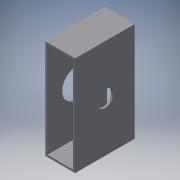
# Autodesk Inventor part: transmition Axle Support
Saved by Autodesk Inventor 2019 (Build 230136000, 136)
## iProperties
Created: 2019-10-21
Part Number: transmition Axle Support
Material: Generic
Document SubType Name: Modeling
Designer: admin
Density: 1 g/cm^3
Appearance: Default
Author: admin
Autodesk Inventor part; units mm, degrees
ref_plane "YZ Plane" through (0, 0, 0) normal (1, 0, 0) x (0, 1, 0)
ref_plane "XZ Plane" through (0, 0, 0) normal (0, 1, 0) x (-1, 0, 0)
ref_plane "XY Plane" through (0, 0, 0) normal (0, 0, 1) x (1, 0, 0)
sketch "Sketch1" plane through (0, 0, 0) normal (0, 0, 1) x (1, 0, 0)
  line L0 (-15, -50) -> (15, -50)
  line L1 (15, -50) -> (15, 50)
  line L2 (15, 50) -> (-15, 50)
  line L3 (-15, 50) -> (-15, -50)
  line L4 (-15, -50) -> (15, 50) construction
  line L5 (15, -50) -> (-15, 50) construction
  line L6 (-13, 48) -> (13, 48)
  line L7 (13, 48) -> (13, -48)
  line L8 (13, -48) -> (-13, -48)
  line L9 (-13, -48) -> (-13, 48)
  point P0 (0, 0)
  dimension "d0" = 30
  dimension "d1" = 100
  dimension "d2" = 2
  constraints: 20 end point, 4 parallel, 2 midpoint, 2 perpendicular, 1 horizontal, 3 other
  measures "d0" distance of L2.end L1.end
  measures "d1" distance of L1.end L0.end
  measures "d2" distance between parallel lines of L2 L6
extrude "Extrusion1" add sketch "Sketch1" along normal blind 60
sketch "Sketch2" plane through (15, -50, 0) normal (1, 0, 0) x (0, 0, -1)
  circle A0 centre (-30, 50) radius 8.3
  line L0 (-30, 100) -> (-30, 50) construction
  line L1 (0, 0) -> (0, 100) projected
  line L2 (0, 100) -> (-60, 100) projected
  line L3 (-30, 50) -> (0, 50) construction
  dimension "d5" = 16.6
  dimension "d11" = 50
  dimension "d12" = 30
  constraints: 4 end point, 1 centre point, 1 horizontal, 1 midpoint, 1 vertical
  measures "d5" diameter of A0
  measures "d11" distance from line of L2 L0.end
  measures "d12" distance from line of L1 L0.end
extrude "Extrusion2" cut sketch "Sketch2" against normal blind 2
sketch "Sketch3" plane through (-13, -48, 0) normal (1, 0, 0) x (0, 0, -1)
  circle A0 centre (-30, 48) radius 8.3 projected
  circle A1 centre (-30, 48) radius 15
  point P0 (0, 48)
  dimension "d8" = 30
  constraints: 1 centre point, 1 coincident
  measures "d8" diameter of A1
extrude "Extrusion3" cut sketch "Sketch3" against normal blind 2 contours A0 | A1
body "Solid1"
